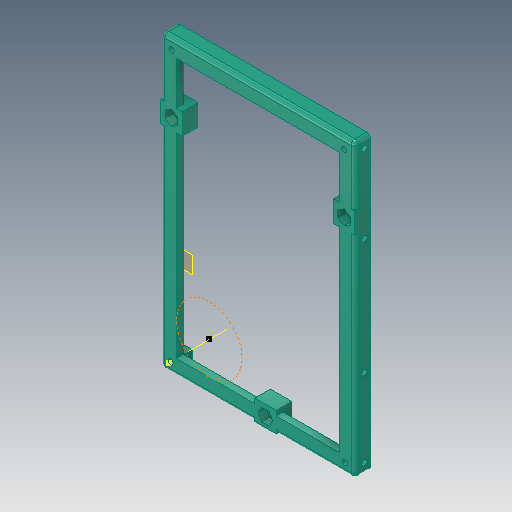
# Autodesk Inventor part: 10_Lid_el_4x2_v2
Saved by Autodesk Inventor 2019 (Build 230136000, 136)
## iProperties
Created: 2019-07-01
Part Number: 10_Lid_el_4x2_v2
Material: Generic
Document SubType Name: Modeling
Designer: diederichbenedict
Density: 1 g/cm^3
Appearance: IPHT_Türkis
Author: diederichbenedict
Autodesk Inventor part; units mm, degrees
ref_plane "YZ Plane" through (0, 0, 0) normal (1, 0, 0) x (0, 1, 0)
ref_plane "XZ Plane" through (0, 0, 0) normal (0, 1, 0) x (-1, 0, 0)
ref_plane "XY Plane" through (0, 0, 0) normal (0, 0, 1) x (1, 0, 0)
ref_plane "Work Plane1" through (0, 41.8, 0) normal (0, 0, 1) x (1, 0, 0)
sketch "Sketch1" plane through (0, 41.8, 0) normal (0, 0, 1) x (1, 0, 0)
  circle A0 centre (0.9, -0.9) radius 1.45 construction
  line L0 (4, -1.5) -> (1.5, -4) construction
  line L1 (4, -1.5) -> (4, 4) construction
  line L2 (4, 4) -> (-2, 4) construction
  arc A1 (-2, 4) -> (-4, 2) centre (-2, 2) ccw construction
  line L3 (-4, 2) -> (-4, -4) construction
  line L4 (-4, -4) -> (1.5, -4) construction
  arc A2 (45.8, 2) -> (43.8, 4) centre (43.8, 2) ccw construction
  line L5 (43.8, 4) -> (37.8, 4) construction
  line L6 (37.8, 4) -> (37.8, -1.5) construction
  line L7 (40.3, -4) -> (45.8, -4) construction
  line L8 (45.8, -4) -> (45.8, 2) construction
  circle A3 centre (40.9, -0.9) radius 1.45 construction
  line L9 (37.8, -40.3) -> (40.3, -37.8) construction
  line L10 (37.8, -40.3) -> (37.8, -45.8) construction
  line L11 (37.8, -45.8) -> (43.8, -45.8) construction
  arc A4 (43.8, -45.8) -> (45.8, -43.8) centre (43.8, -43.8) ccw construction
  line L12 (45.8, -43.8) -> (45.8, -37.8) construction
  line L13 (45.8, -37.8) -> (40.3, -37.8) construction
  circle A5 centre (40.9, -40.9) radius 1.45 construction
  circle A6 centre (0.9, -40.9) radius 1.45 construction
  line L14 (1.5, -37.8) -> (4, -40.3) construction
  line L15 (1.5, -37.8) -> (-4, -37.8) construction
  line L16 (-4, -37.8) -> (-4, -43.8) construction
  arc A7 (-4, -43.8) -> (-2, -45.8) centre (-2, -43.8) ccw construction
  line L17 (-2, -45.8) -> (4, -45.8) construction
  line L18 (4, -45.8) -> (4, -40.3) construction
  line L19 (40.3, -4) -> (37.8, -1.5) construction
  line L20 (-2, 104) -> (93.8, 104)
  line L21 (95.8, 102) -> (95.8, -43.8)
  line L22 (93.8, -45.8) -> (-2, -45.8)
  line L23 (-4, -43.8) -> (-4, 102)
  line L24 (90.3, -37.8) -> (90.3, 96)
  line L25 (87.8, 98.5) -> (4, 98.5)
  line L26 (1.5, 96) -> (1.5, -37.8)
  line L27 (4, -40.3) -> (87.8, -40.3)
  line L28 (87.8, -40.3) -> (90.3, -37.8)
  line L29 (4, -40.3) -> (1.5, -37.8)
  line L30 (4, 98.5) -> (1.5, 96)
  line L31 (90.3, 96) -> (87.8, 98.5)
  arc A8 (95.8, 102) -> (93.8, 104) centre (93.8, 102) ccw
  arc A9 (93.8, -45.8) -> (95.8, -43.8) centre (93.8, -43.8) ccw
  arc A10 (-4, -43.8) -> (-2, -45.8) centre (-2, -43.8) ccw
  arc A11 (-2, 104) -> (-4, 102) centre (-2, 102) ccw
  circle A12 centre (90.8, -40.8) radius 1.4
  circle A13 centre (1, -40.8) radius 1.4
  circle A14 centre (45.9, 54.1) radius 44.4 construction
  line L32 (4, 96) -> (4, -37.8)
  line L33 (4, -37.8) -> (87.8, -37.8)
  line L34 (87.8, -37.8) -> (87.8, 96)
  line L35 (87.8, 96) -> (4, 96)
  circle A15 centre (1.5, 98.5) radius 1.4
  circle A16 centre (90.3, 98.5) radius 1.4
  point P0 (95.8, -45.8)
  point P1 (95.8, 104)
  point P2 (-4, -45.8)
  point P3 (90.3, -40.3)
  point P4 (1.5, -40.3)
  point P5 (40.8, 99)
  dimension "d34" = 99.8
  dimension "d35" = 149.8
  dimension "d36" = 5.5
  dimension "d37" = 2.5
  dimension "d38" = 2.5
  dimension "d39" = 2.5
  dimension "d40" = 2.5
  dimension "d41" = 2.5
  dimension "d42" = 2.5
  dimension "d43" = 2.5
  dimension "d44" = 2.5
  dimension "d45" = 2
  dimension "d46" = 5
  dimension "d47" = 5
  dimension "d48" = 5
  dimension "d49" = 5
  dimension "d50" = 5
  dimension "d51" = 5
  dimension "d57" = 2.8
  dimension "d58" = 2.8
  dimension "d90" = 8
  dimension "d102" = 2.8
  dimension "d103" = 2.8
  constraints: 32 end point, 14 point on line, 11 tangent, 9 centre point, 8 point on circle, 6 parallel, 4 coincident, 3 equal radius, 3 perpendicular, 1 horizontal, 6 other
  measures "d34" distance of point (95.8, -45.8) point (-4, -45.8)
  measures "d35" distance of point (95.8, 104) point (95.8, -45.8)
  measures "d36" distance between parallel lines of L21 L24
  measures "d37" distance of L27.end point (90.3, -40.3)
  measures "d38" distance of L24.start point (90.3, -40.3)
  measures "d39" distance of L27.start point (1.5, -40.3)
  measures "d40" distance of L26.end point (1.5, -40.3)
  measures "d41" distance of L25.end point (1.5, 98.5)
  measures "d42" distance of L26.start point (1.5, 98.5)
  measures "d43" distance of L24.end point (90.3, 98.5)
  measures "d44" distance of L25.start point (90.3, 98.5)
  measures "d45" radius of A8
  measures "d46" distance from line of point (1, -40.8) L23
  measures "d47" distance from line of L22 point (1, -40.8)
  measures "d48" distance from line of L21 point (90.8, -40.8)
  measures "d49" distance from line of L22 point (90.8, -40.8)
  measures "d50" distance from line of L8 point (40.8, 99)
  measures "d51" distance from line of L20 point (40.8, 99)
  measures "d57" diameter of A12
  measures "d58" diameter of A13
  measures "d90" distance between parallel lines of L23 L32
  measures "d102" diameter of A15
  measures "d103" diameter of A16
extrude "Extrusion1" add sketch "Sketch1" along normal blind 8 contours L20 A8 L21 A9 L22 A10 L23 A11 | L28 L27 L29 L26 L30 L25 L31 L24
fillet "Fillet1" radius 2 8 edges at (45.9, -4, 8) (95.2142, -3.4142, 8) (95.8, 70.9, 8) (95.2142, 145.2142, 8) (45.9, 145.8, 8) (-3.4142, 145.2142, 8) (-4, 70.9, 8) (-3.4142, -3.4142, 8)
sketch "Sketch3" plane through (0, 41.8, 8) normal (0, 0, 1) x (1, 0, 0)
  circle A0 centre (20.9, -20.9) radius 16.9 construction
  point P0 (0, -41.8)
  constraints: 1 centre point
chamfer "Chamfer2" distance 4.5 angle 45 2 edges at (4, 70.9, 0) (87.8, 70.9, 0)
sketch "Sketch7" plane through (95.8, -2, 0) normal (1, 0, 0) x (0, 0, -1)
  circle A0 centre (-3.1, 142.8) radius 1.4 projected
  circle A1 centre (-3.1, 3) radius 1.4 projected
  circle A2 centre (-3.1, 43) radius 1.4 projected
  circle A3 centre (-3.1, 102.8) radius 1.4 projected
  point P0 (0, 2)
  point P1 (-3, 101.4036)
  point P2 (-3, 104.1964)
  constraints: 1 vertical alignment
hole "Hole4" at (95.8, 140.8, 3.1) at (95.8, 1, 3.1) at (95.8, 41, 3.1) at (95.8, 100.8, 3.1) direction (-1, 0, 0) diameter 2.8 depth 6.5 tip angle 118
sketch "Sketch9" plane through (87.8, 4, 8) normal (-1, 0, 0) x (0, 0, 1)
  line L0 (-8, 0) -> (-3.5, 0) projected
  line L1 (-3.5, 133.8) -> (-8, 133.8) projected
  line L2 (-3.5, 0) -> (-8, -4.5)
  line L3 (-8, 139.8) -> (-8, -6) projected
  line L4 (-3.5, 0) -> (2.864, 0) construction
  line L5 (-8, -4.5) -> (-8, 0)
  line L6 (-3.5, 133.8) -> (-8, 138.3)
  line L7 (-3.5, 133.8) -> (2.864, 133.8) construction
  line L8 (-8, 138.3) -> (-8, 133.8)
  line L9 (-8, 133.8) -> (-3.5, 133.8)
  point P0 (-8, -4)
  dimension "d91" = 135
  dimension "d92" = 135
  constraints: 14 end point, 3 collinear, 2 equal length, 2 horizontal, 2 point on line
  measures "d91" angle of L2 L4
  measures "d92" angle of L7 L6
extrude "Extrusion3" cut sketch "Sketch9" along normal up to surface (83.8 mm away)
sketch "Sketch11" plane through (0, 41.8, 0) normal (0, 0, -1) x (-1, 0, 0)
  circle A0 centre (-1.5, 68.2461) radius 1.6 projected
  circle A1 centre (-90.3, 68.2461) radius 1.6 projected
  circle A2 centre (-49.8, -40.8) radius 1.6 projected
  line L0 (0.5, -37.8) -> (0.5, 96) projected
  line L1 (-92.3, 96) -> (-92.3, -37.8) projected
  line L2 (-87.8, -37.8) -> (-4, -37.8) projected
  line L3 (4, -43.8) -> (4, 102) projected
  line L4 (-7, 62.7461) -> (4, 62.7461)
  line L5 (4, 62.7461) -> (4, 73.7461)
  line L6 (4, 73.7461) -> (-7, 73.7461)
  line L7 (-7, 73.7461) -> (-7, 62.7461)
  line L8 (-7, 62.7461) -> (4, 73.7461) construction
  line L9 (4, 62.7461) -> (-7, 73.7461) construction
  line L10 (-84.8, 62.7461) -> (-95.8, 62.7461)
  line L11 (-95.8, 62.7461) -> (-95.8, 73.7461)
  line L12 (-95.8, 73.7461) -> (-84.8, 73.7461)
  line L13 (-84.8, 73.7461) -> (-84.8, 62.7461)
  line L14 (-84.8, 62.7461) -> (-95.8, 73.7461) construction
  line L15 (-95.8, 62.7461) -> (-84.8, 73.7461) construction
  line L16 (-55.3, -46.3) -> (-44.3, -46.3)
  line L17 (-44.3, -46.3) -> (-44.3, -35.3)
  line L18 (-44.3, -35.3) -> (-55.3, -35.3)
  line L19 (-55.3, -35.3) -> (-55.3, -46.3)
  line L20 (-55.3, -46.3) -> (-44.3, -35.3) construction
  line L21 (-44.3, -46.3) -> (-55.3, -35.3) construction
  line L22 (2, -45.8) -> (-93.8, -45.8) projected
  line L23 (-44.3, -45.8) -> (-55.3, -45.8)
  point P0 (0, -41.8)
  dimension "d104" = 11
  dimension "d105" = 11
  dimension "d106" = 11
  dimension "d107" = 11
  dimension "d108" = 11
  constraints: 38 end point, 6 midpoint, 6 parallel, 5 point on line, 3 horizontal, 3 perpendicular
  measures "d104" distance of L5.end L4.end
  measures "d105" distance of L11.end L12.end
  measures "d106" distance of L10.end L11.end
  measures "d107" distance of L18.end L17.end
  measures "d108" distance of L17.end L16.end
extrude "Extrusion5" add sketch "Sketch11" against normal up to surface (8 mm away) contours L4 L7 L6 L0 | L0 L6 L3 L4 | L12 L13 L10 L1 | L1 L10 L11 L12 | L19 L18 L17 L2 | L2 L17 L22 L19
sketch "Sketch12" plane through (0, 41.8, 0) normal (0, 0, -1) x (-1, 0, 0)
  circle A0 centre (-1.5, 68.2461) radius 1.6 projected
  circle A1 centre (-90.3, 68.2461) radius 1.6 projected
  circle A2 centre (-49.8, -40.8) radius 1.6 projected
  point P0 (0, -41.8)
extrude "Extrusion6" cut sketch "Sketch12" against normal blind 10
sketch "Sketch13" plane through (0, 41.8, 8) normal (0, 0, 1) x (1, 0, 0)
  circle A0 centre (90.3, 68.2461) radius 1.6 projected
  circle A1 centre (1.5, 68.2461) radius 1.6 projected
  circle A2 centre (49.8, -40.8) radius 1.6 projected
  line L0 (93.55, 70.1224) -> (93.55, 66.3697)
  line L1 (93.55, 66.3697) -> (90.3, 64.4933)
  line L2 (90.3, 64.4933) -> (87.05, 66.3697)
  line L3 (87.05, 66.3697) -> (87.05, 70.1224)
  line L4 (87.05, 70.1224) -> (90.3, 71.9988)
  line L5 (90.3, 71.9988) -> (93.55, 70.1224)
  line L6 (4.75, 70.1224) -> (4.75, 66.3697)
  line L7 (4.75, 66.3697) -> (1.5, 64.4933)
  line L8 (1.5, 64.4933) -> (-1.75, 66.3697)
  line L9 (-1.75, 66.3697) -> (-1.75, 70.1224)
  line L10 (-1.75, 70.1224) -> (1.5, 71.9988)
  line L11 (1.5, 71.9988) -> (4.75, 70.1224)
  line L12 (51.6764, -37.55) -> (53.5528, -40.8)
  line L13 (53.5528, -40.8) -> (51.6764, -44.05)
  line L14 (51.6764, -44.05) -> (47.9236, -44.05)
  line L15 (47.9236, -44.05) -> (46.0472, -40.8)
  line L16 (46.0472, -40.8) -> (47.9236, -37.55)
  line L17 (47.9236, -37.55) -> (51.6764, -37.55)
  line L18 (95.8, 73.7461) -> (95.8, 62.7461) projected
  line L19 (-4, 62.7461) -> (-4, 73.7461) projected
  line L20 (44.3, -35.3) -> (55.3, -35.3) projected
  point P0 (0, -41.8)
  point P1 (90.3, 68.2461)
  point P2 (1.5, 68.2461)
  point P3 (49.8, -40.8)
  dimension "d113" = 6.5
  dimension "d114" = 6.5
  dimension "d115" = 6.5
  constraints: 36 end point, 3 coincident, 3 parallel, 39 other
  measures "d113" distance between parallel lines of L3 L0
  measures "d114" distance between parallel lines of L9 L6
  measures "d115" distance between parallel lines of L15 L12
extrude "Extrusion7" cut sketch "Sketch13" against normal blind 4
equation "\"d38\" = d37"
equation "\"d39\" = d37"
equation "\"d40\" = d39"
equation "\"d41\" = d37"
equation "\"d42\" = d41"
equation "\"d43\" = d37"
equation "\"d44\" = d43"
body "Solid1"
